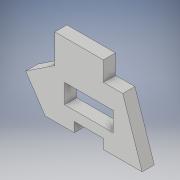
# Autodesk Inventor part: P2-2
Saved by Autodesk Inventor 2017 (Build 210142000, 142)
## iProperties
Created: 2017-02-09
Part Number: P2-2
Material: Generic
Document SubType Name: Modeling
Designer: Schaffel
Density: 1 g/cm^3
Appearance: Default
Author: Schaffel
Autodesk Inventor part; units mm, degrees
ref_plane "YZ Plane" through (0, 0, 0) normal (1, 0, 0) x (0, 1, 0)
ref_plane "XZ Plane" through (0, 0, 0) normal (0, 1, 0) x (-1, 0, 0)
ref_plane "XY Plane" through (0, 0, 0) normal (0, 0, 1) x (1, 0, 0)
sketch "Sketch1" plane through (0, 0, 0) normal (0, 0, 1) x (1, 0, 0)
  line L0 (25.4, 0) -> (0, 38.1)
  line L1 (63.5, 0) -> (25.4, 0)
  line L2 (63.5, 0) -> (63.5, 12.7)
  line L3 (63.5, 12.7) -> (101.6, 12.7)
  line L4 (101.6, 12.7) -> (101.6, 0)
  line L5 (50.8, 25.4) -> (50.8, 50.8)
  line L6 (50.8, 50.8) -> (114.3, 50.8)
  line L7 (114.3, 50.8) -> (114.3, 25.4)
  line L8 (114.3, 25.4) -> (50.8, 25.4)
  line L9 (101.6, 0) -> (152.4, 0)
  line L10 (152.4, 0) -> (127, 76.2)
  line L11 (127, 76.2) -> (101.6, 76.2)
  line L12 (101.6, 76.2) -> (101.6, 101.6)
  line L13 (101.6, 101.6) -> (38.1, 101.6)
  line L14 (38.1, 101.6) -> (38.1, 63.5)
  line L15 (38.1, 63.5) -> (0, 38.1)
  point P0 (0, 0)
  constraints: 32 end point, 6 perpendicular, 3 vertical, 1 horizontal, 1 point on line
extrude "Extrusion1" add sketch "Sketch1" along normal blind 15.875
body "Solid1"
